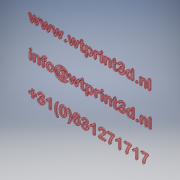
# Autodesk Inventor part: tekst
Saved by Autodesk Inventor 2019.4 (Build 234330000, 330)
## iProperties
Created: 2020-06-08
Part Number: tekst
Material: Generic
Document SubType Name: Modeling
Designer: Jaap Kort
Density: 1 g/cm^3
Appearance: Dark Red
Author: Jaap Kort
Autodesk Inventor part; units mm, degrees
(part 1 of 2)
ref_plane "YZ Plane" through (0, 0, 0) normal (1, 0, 0) x (0, 1, 0)
ref_plane "XZ Plane" through (0, 0, 0) normal (0, 1, 0) x (-1, 0, 0)
ref_plane "XY Plane" through (0, 0, 0) normal (0, 0, 1) x (1, 0, 0)
sketch "Sketch1" plane through (0, 0, 0) normal (0, 0, 1) x (1, 0, 0)
  line L0 (0, 0) -> (85, 0) construction
  line L1 (85, 0) -> (85, 50) construction
  line L2 (85, 50) -> (0, 50) construction
  line L3 (0, 50) -> (0, 0) construction
  line L4 (5.8901, 47.723) -> (80.1344, 47.723) construction
  line L5 (80.1344, 47.723) -> (80.1344, 6.1788) construction
  line L6 (80.1344, 6.1788) -> (5.8901, 6.1788) construction
  line L7 (5.8901, 6.1788) -> (5.8901, 47.723) construction
  line L8 (7.2722, 45.4071) -> (7.887, 43.082)
  line L9 (7.887, 43.082) -> (8.4417, 45.2407)
  spline S0 degree 2 poles (8.4417, 45.2407) (8.5434, 45.5874) (8.6543, 45.8694) (8.964, 46.1329) (9.2275, 46.1329) knots 0 0 0 1 2 3 3 3
  spline S1 degree 2 poles (9.2275, 46.1329) (9.4956, 46.1329) (9.8099, 45.8694) (9.9255, 45.5782) (10.0133, 45.2823) knots 0 0 0 1 2 3 3 3
  line L10 (10.0133, 45.2823) -> (10.5819, 43.082)
  line L11 (10.5819, 43.082) -> (11.2152, 45.4395)
  spline S2 degree 2 poles (11.2152, 45.4395) (11.2753, 45.666) (11.3677, 45.9202) (11.6127, 46.1329) (11.8346, 46.1329) knots 0 0 0 1 2 3 3 3
  spline S3 degree 2 poles (11.8346, 46.1329) (12.0611, 46.1329) (12.3939, 45.8185) (12.3939, 45.6059) knots 0 0 0 1 2 2 2
  spline S4 degree 2 poles (12.3939, 45.6059) (12.3939, 45.4303) (12.2599, 45.0605) knots 0 0 0 1 1 1
  line L12 (12.2599, 45.0605) -> (11.377, 42.4672)
  spline S5 degree 2 poles (11.377, 42.4672) (11.2799, 42.2038) (11.1458, 41.8848) (10.8408, 41.6259) (10.5727, 41.6259) knots 0 0 0 1 2 3 3 3
  spline S6 degree 2 poles (10.5727, 41.6259) (10.2953, 41.6259) (9.981, 41.8987) (9.8377, 42.2823) (9.7637, 42.5366) knots 0 0 0 1 2 3 3 3
  line L13 (9.7637, 42.5366) -> (9.2275, 44.5843)
  line L14 (9.2275, 44.5843) -> (8.7098, 42.5366)
  spline S7 degree 2 poles (8.7098, 42.5366) (8.5942, 42.1159) (8.2938, 41.6259) (7.9009, 41.6259) knots 0 0 0 1 2 2 2
  spline S8 degree 2 poles (7.9009, 41.6259) (7.7021, 41.6259) (7.4201, 41.7831) (7.2352, 42.0651) (7.1197, 42.3887) (7.0734, 42.5227) knots 0 0 0 1 2 3 4 4 4
  line L15 (7.0734, 42.5227) -> (6.2136, 45.0605)
  spline S9 degree 2 poles (6.2136, 45.0605) (6.075, 45.4534) (6.075, 45.6059) knots 0 0 0 1 1 1
  spline S10 degree 2 poles (6.075, 45.6059) (6.075, 45.8139) (6.3939, 46.1329) (6.6343, 46.1329) knots 0 0 0 1 2 2 2
  spline S11 degree 2 poles (6.6343, 46.1329) (6.944, 46.1329) (7.1613, 45.7816) (7.2722, 45.4071) knots 0 0 0 1 2 2 2
  line L16 (13.9286, 45.4071) -> (14.5434, 43.082)
  line L17 (14.5434, 43.082) -> (15.0981, 45.2407)
  spline S12 degree 2 poles (15.0981, 45.2407) (15.1998, 45.5874) (15.3107, 45.8694) (15.6204, 46.1329) (15.8839, 46.1329) knots 0 0 0 1 2 3 3 3
  spline S13 degree 2 poles (15.8839, 46.1329) (16.152, 46.1329) (16.4663, 45.8694) (16.5819, 45.5782) (16.6697, 45.2823) knots 0 0 0 1 2 3 3 3
  line L18 (16.6697, 45.2823) -> (17.2383, 43.082)
  line L19 (17.2383, 43.082) -> (17.8716, 45.4395)
  spline S14 degree 2 poles (17.8716, 45.4395) (17.9317, 45.666) (18.0241, 45.9202) (18.2691, 46.1329) (18.491, 46.1329) knots 0 0 0 1 2 3 3 3
  spline S15 degree 2 poles (18.491, 46.1329) (18.7175, 46.1329) (19.0503, 45.8185) (19.0503, 45.6059) knots 0 0 0 1 2 2 2
  spline S16 degree 2 poles (19.0503, 45.6059) (19.0503, 45.4303) (18.9163, 45.0605) knots 0 0 0 1 1 1
  line L20 (18.9163, 45.0605) -> (18.0334, 42.4672)
  spline S17 degree 2 poles (18.0334, 42.4672) (17.9363, 42.2038) (17.8022, 41.8848) (17.4972, 41.6259) (17.2291, 41.6259) knots 0 0 0 1 2 3 3 3
  spline S18 degree 2 poles (17.2291, 41.6259) (16.9517, 41.6259) (16.6374, 41.8987) (16.4941, 42.2823) (16.4201, 42.5366) knots 0 0 0 1 2 3 3 3
  line L21 (16.4201, 42.5366) -> (15.8839, 44.5843)
  line L22 (15.8839, 44.5843) -> (15.3662, 42.5366)
  spline S19 degree 2 poles (15.3662, 42.5366) (15.2506, 42.1159) (14.9502, 41.6259) (14.5572, 41.6259) knots 0 0 0 1 2 2 2
  spline S20 degree 2 poles (14.5572, 41.6259) (14.3585, 41.6259) (14.0765, 41.7831) (13.8916, 42.0651) (13.776, 42.3887) (13.7298, 42.5227) knots 0 0 0 1 2 3 4 4 4
  line L23 (13.7298, 42.5227) -> (12.87, 45.0605)
  spline S21 degree 2 poles (12.87, 45.0605) (12.7314, 45.4534) (12.7314, 45.6059) knots 0 0 0 1 1 1
  spline S22 degree 2 poles (12.7314, 45.6059) (12.7314, 45.8139) (13.0503, 46.1329) (13.2907, 46.1329) knots 0 0 0 1 2 2 2
  spline S23 degree 2 poles (13.2907, 46.1329) (13.6004, 46.1329) (13.8176, 45.7816) (13.9286, 45.4071) knots 0 0 0 1 2 2 2
  line L24 (20.585, 45.4071) -> (21.1998, 43.082)
  line L25 (21.1998, 43.082) -> (21.7545, 45.2407)
  spline S24 degree 2 poles (21.7545, 45.2407) (21.8562, 45.5874) (21.9671, 45.8694) (22.2768, 46.1329) (22.5403, 46.1329) knots 0 0 0 1 2 3 3 3
  spline S25 degree 2 poles (22.5403, 46.1329) (22.8084, 46.1329) (23.1227, 45.8694) (23.2383, 45.5782) (23.3261, 45.2823) knots 0 0 0 1 2 3 3 3
  line L26 (23.3261, 45.2823) -> (23.8947, 43.082)
  line L27 (23.8947, 43.082) -> (24.528, 45.4395)
  spline S26 degree 2 poles (24.528, 45.4395) (24.5881, 45.666) (24.6805, 45.9202) (24.9255, 46.1329) (25.1474, 46.1329) knots 0 0 0 1 2 3 3 3
  spline S27 degree 2 poles (25.1474, 46.1329) (25.3739, 46.1329) (25.7067, 45.8185) (25.7067, 45.6059) knots 0 0 0 1 2 2 2
  spline S28 degree 2 poles (25.7067, 45.6059) (25.7067, 45.4303) (25.5727, 45.0605) knots 0 0 0 1 1 1
  line L28 (25.5727, 45.0605) -> (24.6898, 42.4672)
  spline S29 degree 2 poles (24.6898, 42.4672) (24.5927, 42.2038) (24.4586, 41.8848) (24.1536, 41.6259) (23.8854, 41.6259) knots 0 0 0 1 2 3 3 3
  spline S30 degree 2 poles (23.8854, 41.6259) (23.6081, 41.6259) (23.2938, 41.8987) (23.1505, 42.2823) (23.0765, 42.5366) knots 0 0 0 1 2 3 3 3
  line L29 (23.0765, 42.5366) -> (22.5403, 44.5843)
  line L30 (22.5403, 44.5843) -> (22.0226, 42.5366)
  spline S31 degree 2 poles (22.0226, 42.5366) (21.907, 42.1159) (21.6066, 41.6259) (21.2136, 41.6259) knots 0 0 0 1 2 2 2
  spline S32 degree 2 poles (21.2136, 41.6259) (21.0149, 41.6259) (20.7329, 41.7831) (20.548, 42.0651) (20.4324, 42.3887) (20.3862, 42.5227) knots 0 0 0 1 2 3 4 4 4
  line L31 (20.3862, 42.5227) -> (19.5264, 45.0605)
  spline S33 degree 2 poles (19.5264, 45.0605) (19.3878, 45.4534) (19.3878, 45.6059) knots 0 0 0 1 1 1
  spline S34 degree 2 poles (19.3878, 45.6059) (19.3878, 45.8139) (19.7067, 46.1329) (19.9471, 46.1329) knots 0 0 0 1 2 2 2
  spline S35 degree 2 poles (19.9471, 46.1329) (20.2568, 46.1329) (20.474, 45.7816) (20.585, 45.4071) knots 0 0 0 1 2 2 2
  spline S36 degree 2 poles (27.2044, 41.6259) (26.927, 41.6259) (26.5249, 41.9865) (26.5249, 42.3054) knots 0 0 0 1 2 2 2
  spline S37 degree 2 poles (26.5249, 42.3054) (26.5249, 42.5736) (26.9086, 42.9665) (27.1905, 42.9665) knots 0 0 0 1 2 2 2
  spline S38 degree 2 poles (27.1905, 42.9665) (27.4725, 42.9665) (27.87, 42.5782) (27.87, 42.3054) knots 0 0 0 1 2 2 2
  spline S39 degree 2 poles (27.87, 42.3054) (27.87, 41.9911) (27.4725, 41.6259) (27.2044, 41.6259) knots 0 0 0 1 2 2 2
  line L32 (29.8069, 45.4071) -> (30.4217, 43.082)
  line L33 (30.4217, 43.082) -> (30.9764, 45.2407)
  spline S40 degree 2 poles (30.9764, 45.2407) (31.078, 45.5874) (31.189, 45.8694) (31.4987, 46.1329) (31.7622, 46.1329) knots 0 0 0 1 2 3 3 3
  spline S41 degree 2 poles (31.7622, 46.1329) (32.0303, 46.1329) (32.3446, 45.8694) (32.4602, 45.5782) (32.548, 45.2823) knots 0 0 0 1 2 3 3 3
  line L34 (32.548, 45.2823) -> (33.1166, 43.082)
  line L35 (33.1166, 43.082) -> (33.7499, 45.4395)
  spline S42 degree 2 poles (33.7499, 45.4395) (33.8099, 45.666) (33.9024, 45.9202) (34.1474, 46.1329) (34.3693, 46.1329) knots 0 0 0 1 2 3 3 3
  spline S43 degree 2 poles (34.3693, 46.1329) (34.5958, 46.1329) (34.9286, 45.8185) (34.9286, 45.6059) knots 0 0 0 1 2 2 2
  spline S44 degree 2 poles (34.9286, 45.6059) (34.9286, 45.4303) (34.7945, 45.0605) knots 0 0 0 1 1 1
  line L36 (34.7945, 45.0605) -> (33.9116, 42.4672)
  spline S45 degree 2 poles (33.9116, 42.4672) (33.8146, 42.2038) (33.6805, 41.8848) (33.3754, 41.6259) (33.1073, 41.6259) knots 0 0 0 1 2 3 3 3
  spline S46 degree 2 poles (33.1073, 41.6259) (32.83, 41.6259) (32.5156, 41.8987) (32.3723, 42.2823) (32.2984, 42.5366) knots 0 0 0 1 2 3 3 3
  line L37 (32.2984, 42.5366) -> (31.7622, 44.5843)
  line L38 (31.7622, 44.5843) -> (31.2445, 42.5366)
  spline S47 degree 2 poles (31.2445, 42.5366) (31.1289, 42.1159) (30.8284, 41.6259) (30.4355, 41.6259) knots 0 0 0 1 2 2 2
  spline S48 degree 2 poles (30.4355, 41.6259) (30.2368, 41.6259) (29.9548, 41.7831) (29.7699, 42.0651) (29.6543, 42.3887) (29.6081, 42.5227) knots 0 0 0 1 2 3 4 4 4
  line L39 (29.6081, 42.5227) -> (28.7483, 45.0605)
  spline S49 degree 2 poles (28.7483, 45.0605) (28.6096, 45.4534) (28.6096, 45.6059) knots 0 0 0 1 1 1
  spline S50 degree 2 poles (28.6096, 45.6059) (28.6096, 45.8139) (28.9286, 46.1329) (29.169, 46.1329) knots 0 0 0 1 2 2 2
  spline S51 degree 2 poles (29.169, 46.1329) (29.4787, 46.1329) (29.6959, 45.7816) (29.8069, 45.4071) knots 0 0 0 1 2 2 2
  line L40 (35.7791, 46.0404) -> (35.8115, 46.0404)
  line L41 (35.8115, 46.0404) -> (35.8115, 46.6044)
  spline S52 degree 2 poles (35.8115, 46.6044) (35.8115, 46.8679) (35.8392, 47.1776) (35.9317, 47.3301) knots 0 0 0 1 2 2 2
  spline S53 degree 2 poles (35.9317, 47.3301) (35.9825, 47.4272) (36.2599, 47.5843) (36.4263, 47.5843) knots 0 0 0 1 2 2 2
  spline S54 degree 2 poles (36.4263, 47.5843) (36.662, 47.5843) (36.8515, 47.4087) knots 0 0 0 1 1 1
  spline S55 degree 2 poles (36.8515, 47.4087) (36.981, 47.2885) (37.0457, 46.9603) (37.0457, 46.6876) knots 0 0 0 1 2 2 2
  line L42 (37.0457, 46.6876) -> (37.0457, 46.0404)
  line L43 (37.0457, 46.0404) -> (37.3554, 46.0404)
  spline S56 degree 2 poles (37.3554, 46.0404) (37.6143, 46.0404) (37.9055, 45.7769) (37.9055, 45.5782) knots 0 0 0 1 2 2 2
  spline S57 degree 2 poles (37.9055, 45.5782) (37.9055, 45.3101) (37.4987, 45.1067) (37.1613, 45.1067) knots 0 0 0 1 2 2 2
  line L44 (37.1613, 45.1067) -> (37.0457, 45.1067)
  line L45 (37.0457, 45.1067) -> (37.0457, 43.2207)
  spline S58 degree 2 poles (37.0457, 43.2207) (37.0457, 42.9711) (37.078, 42.7307) (37.189, 42.6105) (37.323, 42.6105) knots 0 0 0 1 2 3 3 3
  spline S59 degree 2 poles (37.323, 42.6105) (37.4109, 42.6105) (37.7344, 42.6752) (37.8269, 42.6752) knots 0 0 0 1 2 2 2
  spline S60 degree 2 poles (37.8269, 42.6752) (37.9933, 42.6752) (38.2475, 42.421) (38.2475, 42.2407) knots 0 0 0 1 2 2 2
  spline S61 degree 2 poles (38.2475, 42.2407) (38.2475, 41.931) (37.6189, 41.6259) (37.0734, 41.6259) knots 0 0 0 1 2 2 2
  spline S62 degree 2 poles (37.0734, 41.6259) (36.5465, 41.6259) (35.9825, 41.9911) (35.8115, 42.629) (35.8115, 43.1375) knots 0 0 0 1 2 3 3 3
  line L46 (35.8115, 43.1375) -> (35.8115, 45.1067)
  line L47 (35.8115, 45.1067) -> (35.756, 45.1067)
  spline S63 degree 2 poles (35.756, 45.1067) (35.4879, 45.1067) (35.1967, 45.3702) (35.1967, 45.5782) knots 0 0 0 1 2 2 2
  spline S64 degree 2 poles (35.1967, 45.5782) (35.1967, 45.7816) (35.5018, 46.0404) (35.7791, 46.0404) knots 0 0 0 1 2 2 2
  line L48 (39.6851, 45.4534) -> (39.6851, 45.4071)
  spline S65 degree 2 poles (39.6851, 45.4071) (39.8469, 45.7585) (40.5311, 46.1236) (40.9656, 46.1236) knots 0 0 0 1 2 2 2
  spline S66 degree 2 poles (40.9656, 46.1236) (41.4787, 46.1236) (42.3523, 45.5874) (42.8515, 44.5751) (42.8515, 43.891) knots 0 0 0 1 2 3 3 3
  spline S67 degree 2 poles (42.8515, 43.891) (42.8515, 43.3825) (42.565, 42.5273) (42.0565, 41.9403) (41.3631, 41.6259) (40.9656, 41.6259) knots 0 0 0 1 2 3 4 4 4
  spline S68 degree 2 poles (40.9656, 41.6259) (40.4802, 41.6259) (39.8284, 42.0096) (39.6851, 42.3471) knots 0 0 0 1 2 2 2
  line L49 (39.6851, 42.3471) -> (39.6851, 40.8263)
  spline S69 degree 2 poles (39.6851, 40.8263) (39.6851, 40.0404) (39.0888, 40.0404) knots 0 0 0 1 1 1
  spline S70 degree 2 poles (39.0888, 40.0404) (38.7329, 40.0404) (38.5064, 40.4657) (38.5064, 40.8355) knots 0 0 0 1 2 2 2
  line L50 (38.5064, 40.8355) -> (38.5064, 45.4441)
  spline S71 degree 2 poles (38.5064, 45.4441) (38.5064, 45.7816) (38.8161, 46.1329) (39.0888, 46.1329) knots 0 0 0 1 2 2 2
  spline S72 degree 2 poles (39.0888, 46.1329) (39.3523, 46.1329) (39.6851, 45.7723) (39.6851, 45.4534) knots 0 0 0 1 2 2 2
  spline S73 degree 2 poles (41.6127, 43.9002) (41.6127, 44.3024) (41.3723, 44.8709) (40.9517, 45.1714) (40.7021, 45.1714) knots 0 0 0 1 2 3 3 3
  spline S74 degree 2 poles (40.7021, 45.1714) (40.2999, 45.1714) (39.736, 44.5242) (39.736, 43.8817) knots 0 0 0 1 2 2 2
  spline S75 degree 2 poles (39.736, 43.8817) (39.736, 43.2669) (40.2953, 42.6105) (40.7021, 42.6105) knots 0 0 0 1 2 2 2
  spline S76 degree 2 poles (40.7021, 42.6105) (40.9425, 42.6105) (41.3539, 42.8925) (41.6127, 43.4749) (41.6127, 43.9002) knots 0 0 0 1 2 3 3 3
  line L51 (44.8762, 43.2531) -> (44.8762, 42.3609)
  spline S77 degree 2 poles (44.8762, 42.3609) (44.8762, 42.0004) (44.5249, 41.6259) (44.2522, 41.6259) knots 0 0 0 1 2 2 2
  spline S78 degree 2 poles (44.2522, 41.6259) (43.9841, 41.6259) (43.642, 42.005) (43.642, 42.3609) knots 0 0 0 1 2 2 2
  line L52 (43.642, 42.3609) -> (43.642, 45.3332)
  spline S79 degree 2 poles (43.642, 45.3332) (43.642, 46.1329) (44.2475, 46.1329) knots 0 0 0 1 1 1
  spline S80 degree 2 poles (44.2475, 46.1329) (44.5572, 46.1329) (44.8254, 45.7446) (44.83, 45.4719) knots 0 0 0 1 2 2 2
  spline S81 degree 2 poles (44.83, 45.4719) (44.8854, 45.7677) (45.32, 46.1329) (45.6898, 46.1329) knots 0 0 0 1 2 2 2
  spline S82 degree 2 poles (45.6898, 46.1329) (46.0457, 46.1329) (46.7437, 45.7631) (46.7437, 45.4395) knots 0 0 0 1 2 2 2
  spline S83 degree 2 poles (46.7437, 45.4395) (46.7437, 45.2084) (46.4247, 44.9079) (46.2352, 44.9079) knots 0 0 0 1 2 2 2
  spline S84 degree 2 poles (46.2352, 44.9079) (46.1613, 44.9079) (45.7129, 45.0512) (45.5511, 45.0512) knots 0 0 0 1 2 2 2
  spline S85 degree 2 poles (45.5511, 45.0512) (45.3477, 45.0512) (45.0888, 44.8386) (44.9363, 44.3856) (44.8762, 43.7384) (44.8762, 43.2531) knots 0 0 0 1 2 3 4 4 4
  line L53 (48.4725, 45.4487) -> (48.4725, 42.3609)
  spline S86 degree 2 poles (48.4725, 42.3609) (48.4725, 42.005) (48.1212, 41.6259) (47.8485, 41.6259) knots 0 0 0 1 2 2 2
  spline S87 degree 2 poles (47.8485, 41.6259) (47.5757, 41.6259) (47.2383, 42.0142) (47.2383, 42.3609) knots 0 0 0 1 2 2 2
  line L54 (47.2383, 42.3609) -> (47.2383, 45.4164)
  spline S88 degree 2 poles (47.2383, 45.4164) (47.2383, 45.7631) (47.5757, 46.1329) (47.8485, 46.1329) knots 0 0 0 1 2 2 2
  spline S89 degree 2 poles (47.8485, 46.1329) (48.1212, 46.1329) (48.4725, 45.7631) (48.4725, 45.4487) knots 0 0 0 1 2 2 2
  spline S90 degree 2 poles (47.8623, 46.4703) (47.6081, 46.4703) (47.2383, 46.7893) (47.2383, 47.0759) knots 0 0 0 1 2 2 2
  spline S91 degree 2 poles (47.2383, 47.0759) (47.2383, 47.3393) (47.6127, 47.6768) (47.8623, 47.6768) knots 0 0 0 1 2 2 2
  spline S92 degree 2 poles (47.8623, 47.6768) (48.0981, 47.6768) (48.4725, 47.3671) (48.4725, 47.0759) knots 0 0 0 1 2 2 2
  spline S93 degree 2 poles (48.4725, 47.0759) (48.4725, 46.7939) (48.1073, 46.4703) (47.8623, 46.4703) knots 0 0 0 1 2 2 2
  line L55 (50.5989, 45.4672) -> (50.5989, 45.421)
  spline S94 degree 2 poles (50.5989, 45.421) (50.7375, 45.7677) (51.4448, 46.1329) (51.9024, 46.1329) knots 0 0 0 1 2 2 2
  spline S95 degree 2 poles (51.9024, 46.1329) (52.3462, 46.1329) (53.0534, 45.7446) (53.2291, 45.3887) knots 0 0 0 1 2 2 2
  spline S96 degree 2 poles (53.2291, 45.3887) (53.34, 45.1806) (53.4047, 44.7045) (53.4047, 44.3486) knots 0 0 0 1 2 2 2
  line L56 (53.4047, 44.3486) -> (53.4047, 42.3609)
  spline S97 degree 2 poles (53.4047, 42.3609) (53.4047, 42.005) (53.0673, 41.6259) (52.7945, 41.6259) knots 0 0 0 1 2 2 2
  spline S98 degree 2 poles (52.7945, 41.6259) (52.5172, 41.6259) (52.1751, 42.0142) (52.1751, 42.3609) knots 0 0 0 1 2 2 2
  line L57 (52.1751, 42.3609) -> (52.1751, 44.1406)
  spline S99 degree 2 poles (52.1751, 44.1406) (52.1751, 44.6491) (51.9116, 45.1483) (51.5234, 45.1483) knots 0 0 0 1 2 2 2
  spline S100 degree 2 poles (51.5234, 45.1483) (51.2645, 45.1483) (50.8392, 44.8386) (50.7237, 44.5289) knots 0 0 0 1 2 2 2
  spline S101 degree 2 poles (50.7237, 44.5289) (50.6636, 44.344) (50.6636, 43.7014) knots 0 0 0 1 1 1
  line L58 (50.6636, 43.7014) -> (50.6636, 42.3609)
  spline S102 degree 2 poles (50.6636, 42.3609) (50.6636, 42.0004) (50.3169, 41.6259) (50.0395, 41.6259) knots 0 0 0 1 2 2 2
  spline S103 degree 2 poles (50.0395, 41.6259) (49.7714, 41.6259) (49.4294, 42.0142) (49.4294, 42.3609) knots 0 0 0 1 2 2 2
  line L59 (49.4294, 42.3609) -> (49.4294, 45.4487)
  spline S104 degree 2 poles (49.4294, 45.4487) (49.4294, 45.7816) (49.7391, 46.1329) (50.0072, 46.1329) knots 0 0 0 1 2 2 2
  spline S105 degree 2 poles (50.0072, 46.1329) (50.1736, 46.1329) (50.4417, 45.9757) (50.5989, 45.6706) (50.5989, 45.4672) knots 0 0 0 1 2 3 3 3
  line L60 (54.5511, 46.0404) -> (54.5834, 46.0404)
  line L61 (54.5834, 46.0404) -> (54.5834, 46.6044)
  spline S106 degree 2 poles (54.5834, 46.6044) (54.5834, 46.8679) (54.6112, 47.1776) (54.7036, 47.3301) knots 0 0 0 1 2 2 2
  spline S107 degree 2 poles (54.7036, 47.3301) (54.7545, 47.4272) (55.0318, 47.5843) (55.1982, 47.5843) knots 0 0 0 1 2 2 2
  spline S108 degree 2 poles (55.1982, 47.5843) (55.434, 47.5843) (55.6235, 47.4087) knots 0 0 0 1 1 1
  spline S109 degree 2 poles (55.6235, 47.4087) (55.7529, 47.2885) (55.8176, 46.9603) (55.8176, 46.6876) knots 0 0 0 1 2 2 2
  line L62 (55.8176, 46.6876) -> (55.8176, 46.0404)
  line L63 (55.8176, 46.0404) -> (56.1274, 46.0404)
  spline S110 degree 2 poles (56.1274, 46.0404) (56.3862, 46.0404) (56.6774, 45.7769) (56.6774, 45.5782) knots 0 0 0 1 2 2 2
  spline S111 degree 2 poles (56.6774, 45.5782) (56.6774, 45.3101) (56.2707, 45.1067) (55.9332, 45.1067) knots 0 0 0 1 2 2 2
  line L64 (55.9332, 45.1067) -> (55.8176, 45.1067)
  line L65 (55.8176, 45.1067) -> (55.8176, 43.2207)
  spline S112 degree 2 poles (55.8176, 43.2207) (55.8176, 42.9711) (55.85, 42.7307) (55.9609, 42.6105) (56.095, 42.6105) knots 0 0 0 1 2 3 3 3
  spline S113 degree 2 poles (56.095, 42.6105) (56.1828, 42.6105) (56.5064, 42.6752) (56.5989, 42.6752) knots 0 0 0 1 2 2 2
  spline S114 degree 2 poles (56.5989, 42.6752) (56.7653, 42.6752) (57.0195, 42.421) (57.0195, 42.2407) knots 0 0 0 1 2 2 2
  spline S115 degree 2 poles (57.0195, 42.2407) (57.0195, 41.931) (56.3908, 41.6259) (55.8454, 41.6259) knots 0 0 0 1 2 2 2
  spline S116 degree 2 poles (55.8454, 41.6259) (55.3184, 41.6259) (54.7545, 41.9911) (54.5834, 42.629) (54.5834, 43.1375) knots 0 0 0 1 2 3 3 3
  line L66 (54.5834, 43.1375) -> (54.5834, 45.1067)
  line L67 (54.5834, 45.1067) -> (54.528, 45.1067)
  spline S117 degree 2 poles (54.528, 45.1067) (54.2599, 45.1067) (53.9687, 45.3702) (53.9687, 45.5782) knots 0 0 0 1 2 2 2
  spline S118 degree 2 poles (53.9687, 45.5782) (53.9687, 45.7816) (54.2737, 46.0404) (54.5511, 46.0404) knots 0 0 0 1 2 2 2
  spline S119 degree 2 poles (59.0303, 45.3517) (59.3585, 45.3517) (59.83, 45.7307) (59.83, 46.0913) knots 0 0 0 1 2 2 2
  spline S120 degree 2 poles (59.83, 46.0913) (59.83, 46.3548) (59.4602, 46.743) (59.1458, 46.743) knots 0 0 0 1 2 2 2
  spline S121 degree 2 poles (59.1458, 46.743) (58.924, 46.743) (58.6466, 46.6229) (58.4895, 46.4333) (58.3138, 46.0543) (58.263, 45.9434) knots 0 0 0 1 2 3 4 4 4
  spline S122 degree 2 poles (58.263, 45.9434) (58.2121, 45.8278) (57.9671, 45.7169) (57.8146, 45.7169) knots 0 0 0 1 2 2 2
  spline S123 degree 2 poles (57.8146, 45.7169) (57.6204, 45.7169) (57.3107, 46.0219) (57.3107, 46.2669) knots 0 0 0 1 2 2 2
  spline S124 degree 2 poles (57.3107, 46.2669) (57.3107, 46.4934) (57.5742, 46.9695) (58.0734, 47.3948) (58.8038, 47.6537) (59.2522, 47.6537) knots 0 0 0 1 2 3 4 4 4
  spline S125 degree 2 poles (59.2522, 47.6537) (59.6451, 47.6537) (60.3015, 47.4364) (60.7915, 47.0204) (61.0411, 46.4749) (61.0411, 46.1606) knots 0 0 0 1 2 3 4 4 4
  spline S126 degree 2 poles (61.0411, 46.1606) (61.0411, 45.7492) (60.6805, 45.1529) (60.3847, 44.9541) knots 0 0 0 1 2 2 2
  spline S127 degree 2 poles (60.3847, 44.9541) (60.6574, 44.8432) (61.0965, 44.3994) (61.3184, 43.8586) (61.3184, 43.5443) knots 0 0 0 1 2 3 3 3
  spline S128 degree 2 poles (61.3184, 43.5443) (61.3184, 43.1745) (61.018, 42.4765) (60.4401, 41.931) (59.6451, 41.6259) (59.169, 41.6259) knots 0 0 0 1 2 3 4 4 4
  spline S129 degree 2 poles (59.169, 41.6259) (58.679, 41.6259) (57.9024, 41.9773) (57.4032, 42.5042) (57.1443, 43.0728) (57.1443, 43.2669) knots 0 0 0 1 2 3 4 4 4
  spline S130 degree 2 poles (57.1443, 43.2669) (57.1443, 43.5304) (57.4864, 43.854) (57.7406, 43.854) knots 0 0 0 1 2 2 2
  spline S131 degree 2 poles (57.7406, 43.854) (57.8747, 43.854) (58.1197, 43.6922) (58.1659, 43.5489) knots 0 0 0 1 2 2 2
  spline S132 degree 2 poles (58.1659, 43.5489) (58.36, 43.0497) (58.7899, 42.5597) (59.1782, 42.5597) knots 0 0 0 1 2 2 2
  spline S133 degree 2 poles (59.1782, 42.5597) (59.4001, 42.5597) (59.8069, 42.7769) (60.0796, 43.2115) (60.0796, 43.4981) knots 0 0 0 1 2 3 3 3
  spline S134 degree 2 poles (60.0796, 43.4981) (60.0796, 43.9233) (59.622, 44.3948) (59.2152, 44.3948) knots 0 0 0 1 2 2 2
  spline S135 degree 2 poles (59.2152, 44.3948) (59.1458, 44.3948) (58.8177, 44.3625) (58.7622, 44.3625) knots 0 0 0 1 2 2 2
  spline S136 degree 2 poles (58.7622, 44.3625) (58.5126, 44.3625) (58.226, 44.6213) (58.226, 44.8524) knots 0 0 0 1 2 2 2
  spline S137 degree 2 poles (58.226, 44.8524) (58.226, 45.0789) (58.5634, 45.3517) (58.8685, 45.3517) knots 0 0 0 1 2 2 2
  line L68 (58.8685, 45.3517) -> (59.0303, 45.3517)
  line L69 (65.0996, 42.3193) -> (65.0996, 42.3378)
  spline S138 degree 2 poles (65.0996, 42.3378) (65.0257, 42.1159) (64.5865, 41.7924) (64.0734, 41.6259) (63.7683, 41.6259) knots 0 0 0 1 2 3 3 3
  spline S139 degree 2 poles (63.7683, 41.6259) (63.3616, 41.6259) (62.6774, 41.968) (62.1782, 42.5967) (61.924, 43.4333) (61.924, 43.9233) knots 0 0 0 1 2 3 4 4 4
  spline S140 degree 2 poles (61.924, 43.9233) (61.924, 44.9541) (62.9455, 46.1236) (63.7868, 46.1236) knots 0 0 0 1 2 2 2
  spline S141 degree 2 poles (63.7868, 46.1236) (64.2676, 46.1236) (64.9332, 45.7908) (65.0996, 45.4811) knots 0 0 0 1 2 2 2
  line L70 (65.0996, 45.4811) -> (65.0996, 46.9788)
  spline S142 degree 2 poles (65.0996, 46.9788) (65.0996, 47.3347) (65.4047, 47.723) (65.6913, 47.723) knots 0 0 0 1 2 2 2
  spline S143 degree 2 poles (65.6913, 47.723) (65.9687, 47.723) (66.2784, 47.3625) (66.2784, 47.0343) knots 0 0 0 1 2 2 2
  line L71 (66.2784, 47.0343) -> (66.2784, 42.3193)
  spline S144 degree 2 poles (66.2784, 42.3193) (66.2784, 41.9819) (65.9502, 41.6259) (65.6913, 41.6259) knots 0 0 0 1 2 2 2
  spline S145 degree 2 poles (65.6913, 41.6259) (65.4324, 41.6259) (65.0996, 41.9911) (65.0996, 42.3193) knots 0 0 0 1 2 2 2
  spline S146 degree 2 poles (63.1628, 43.8863) (63.1628, 43.4657) (63.417, 42.8925) (63.8469, 42.6105) (64.0965, 42.6105) knots 0 0 0 1 2 3 3 3
  spline S147 degree 2 poles (64.0965, 42.6105) (64.3554, 42.6105) (64.7807, 42.8786) (65.0395, 43.4518) (65.0395, 43.8863) knots 0 0 0 1 2 3 3 3
  spline S148 degree 2 poles (65.0395, 43.8863) (65.0395, 44.2931) (64.7807, 44.8756) (64.3462, 45.1714) (64.0919, 45.1714) knots 0 0 0 1 2 3 3 3
  spline S149 degree 2 poles (64.0919, 45.1714) (63.8238, 45.1714) (63.4032, 44.8663) (63.1628, 44.2839) (63.1628, 43.8863) knots 0 0 0 1 2 3 3 3
  spline S150 degree 2 poles (68.0811, 41.6259) (67.8038, 41.6259) (67.4016, 41.9865) (67.4016, 42.3054) knots 0 0 0 1 2 2 2
  spline S151 degree 2 poles (67.4016, 42.3054) (67.4016, 42.5736) (67.7853, 42.9665) (68.0673, 42.9665) knots 0 0 0 1 2 2 2
  spline S152 degree 2 poles (68.0673, 42.9665) (68.3492, 42.9665) (68.7468, 42.5782) (68.7468, 42.3054) knots 0 0 0 1 2 2 2
  spline S153 degree 2 poles (68.7468, 42.3054) (68.7468, 41.9911) (68.3492, 41.6259) (68.0811, 41.6259) knots 0 0 0 1 2 2 2
  line L72 (70.9933, 45.4672) -> (70.9933, 45.421)
  spline S154 degree 2 poles (70.9933, 45.421) (71.132, 45.7677) (71.8392, 46.1329) (72.2968, 46.1329) knots 0 0 0 1 2 2 2
  spline S155 degree 2 poles (72.2968, 46.1329) (72.7406, 46.1329) (73.4479, 45.7446) (73.6235, 45.3887) knots 0 0 0 1 2 2 2
  spline S156 degree 2 poles (73.6235, 45.3887) (73.7344, 45.1806) (73.7992, 44.7045) (73.7992, 44.3486) knots 0 0 0 1 2 2 2
  line L73 (73.7992, 44.3486) -> (73.7992, 42.3609)
  spline S157 degree 2 poles (73.7992, 42.3609) (73.7992, 42.005) (73.4617, 41.6259) (73.189, 41.6259) knots 0 0 0 1 2 2 2
  spline S158 degree 2 poles (73.189, 41.6259) (72.9116, 41.6259) (72.5696, 42.0142) (72.5696, 42.3609) knots 0 0 0 1 2 2 2
  line L74 (72.5696, 42.3609) -> (72.5696, 44.1406)
  spline S159 degree 2 poles (72.5696, 44.1406) (72.5696, 44.6491) (72.3061, 45.1483) (71.9178, 45.1483) knots 0 0 0 1 2 2 2
  spline S160 degree 2 poles (71.9178, 45.1483) (71.6589, 45.1483) (71.2337, 44.8386) (71.1181, 44.5289) knots 0 0 0 1 2 2 2
  spline S161 degree 2 poles (71.1181, 44.5289) (71.058, 44.344) (71.058, 43.7014) knots 0 0 0 1 1 1
  line L75 (71.058, 43.7014) -> (71.058, 42.3609)
  spline S162 degree 2 poles (71.058, 42.3609) (71.058, 42.0004) (70.7113, 41.6259) (70.434, 41.6259) knots 0 0 0 1 2 2 2
  spline S163 degree 2 poles (70.434, 41.6259) (70.1659, 41.6259) (69.8238, 42.0142) (69.8238, 42.3609) knots 0 0 0 1 2 2 2
  line L76 (69.8238, 42.3609) -> (69.8238, 45.4487)
  spline S164 degree 2 poles (69.8238, 45.4487) (69.8238, 45.7816) (70.1335, 46.1329) (70.4016, 46.1329) knots 0 0 0 1 2 2 2
  spline S165 degree 2 poles (70.4016, 46.1329) (70.568, 46.1329) (70.8361, 45.9757) (70.9933, 45.6706) (70.9933, 45.4672) knots 0 0 0 1 2 3 3 3
  line L77 (74.8022, 42.3609) -> (74.8022, 46.9927)
  spline S166 degree 2 poles (74.8022, 46.9927) (74.8022, 47.344) (75.1304, 47.723) (75.4124, 47.723) knots 0 0 0 1 2 2 2
  spline S167 degree 2 poles (75.4124, 47.723) (75.6944, 47.723) (76.0364, 47.3486) (76.0364, 46.9927) knots 0 0 0 1 2 2 2
  line L78 (76.0364, 46.9927) -> (76.0364, 42.3609)
  spline S168 degree 2 poles (76.0364, 42.3609) (76.0364, 42.0004) (75.6898, 41.6259) (75.4124, 41.6259) knots 0 0 0 1 2 2 2
  spline S169 degree 2 poles (75.4124, 41.6259) (75.1397, 41.6259) (74.8022, 42.0142) (74.8022, 42.3609) knots 0 0 0 1 2 2 2
  line L79 (7.679, 26.418) -> (7.679, 23.3301)
  spline S170 degree 2 poles (7.679, 23.3301) (7.679, 22.9742) (7.3277, 22.5952) (7.0549, 22.5952) knots 0 0 0 1 2 2 2
  spline S171 degree 2 poles (7.0549, 22.5952) (6.7822, 22.5952) (6.4448, 22.9835) (6.4448, 23.3301) knots 0 0 0 1 2 2 2
  line L80 (6.4448, 23.3301) -> (6.4448, 26.3856)
  spline S172 degree 2 poles (6.4448, 26.3856) (6.4448, 26.7323) (6.7822, 27.1021) (7.0549, 27.1021) knots 0 0 0 1 2 2 2
  spline S173 degree 2 poles (7.0549, 27.1021) (7.3277, 27.1021) (7.679, 26.7323) (7.679, 26.418) knots 0 0 0 1 2 2 2
  spline S174 degree 2 poles (7.0688, 27.4395) (6.8146, 27.4395) (6.4448, 27.7585) (6.4448, 28.0451) knots 0 0 0 1 2 2 2
  spline S175 degree 2 poles (6.4448, 28.0451) (6.4448, 28.3086) (6.8192, 28.646) (7.0688, 28.646) knots 0 0 0 1 2 2 2
  spline S176 degree 2 poles (7.0688, 28.646) (7.3046, 28.646) (7.679, 28.3363) (7.679, 28.0451) knots 0 0 0 1 2 2 2
  spline S177 degree 2 poles (7.679, 28.0451) (7.679, 27.7631) (7.3138, 27.4395) (7.0688, 27.4395) knots 0 0 0 1 2 2 2
  line L81 (9.8053, 26.4365) -> (9.8053, 26.3902)
  spline S178 degree 2 poles (9.8053, 26.3902) (9.944, 26.7369) (10.6512, 27.1021) (11.1089, 27.1021) knots 0 0 0 1 2 2 2
  spline S179 degree 2 poles (11.1089, 27.1021) (11.5526, 27.1021) (12.2599, 26.7138) (12.4355, 26.3579) knots 0 0 0 1 2 2 2
  spline S180 degree 2 poles (12.4355, 26.3579) (12.5465, 26.1499) (12.6112, 25.6737) (12.6112, 25.3178) knots 0 0 0 1 2 2 2
  line L82 (12.6112, 25.3178) -> (12.6112, 23.3301)
  spline S181 degree 2 poles (12.6112, 23.3301) (12.6112, 22.9742) (12.2737, 22.5952) (12.001, 22.5952) knots 0 0 0 1 2 2 2
  spline S182 degree 2 poles (12.001, 22.5952) (11.7237, 22.5952) (11.3816, 22.9835) (11.3816, 23.3301) knots 0 0 0 1 2 2 2
  line L83 (11.3816, 23.3301) -> (11.3816, 25.1098)
  spline S183 degree 2 poles (11.3816, 25.1098) (11.3816, 25.6183) (11.1181, 26.1175) (10.7298, 26.1175) knots 0 0 0 1 2 2 2
  spline S184 degree 2 poles (10.7298, 26.1175) (10.471, 26.1175) (10.0457, 25.8078) (9.9301, 25.4981) knots 0 0 0 1 2 2 2
  spline S185 degree 2 poles (9.9301, 25.4981) (9.87, 25.3132) (9.87, 24.6707) knots 0 0 0 1 1 1
  line L84 (9.87, 24.6707) -> (9.87, 23.3301)
  spline S186 degree 2 poles (9.87, 23.3301) (9.87, 22.9696) (9.5233, 22.5952) (9.246, 22.5952) knots 0 0 0 1 2 2 2
  spline S187 degree 2 poles (9.246, 22.5952) (8.9779, 22.5952) (8.6358, 22.9835) (8.6358, 23.3301) knots 0 0 0 1 2 2 2
  line L85 (8.6358, 23.3301) -> (8.6358, 26.418)
  spline S188 degree 2 poles (8.6358, 26.418) (8.6358, 26.7508) (8.9455, 27.1021) (9.2136, 27.1021) knots 0 0 0 1 2 2 2
  spline S189 degree 2 poles (9.2136, 27.1021) (9.3801, 27.1021) (9.6482, 26.9449) (9.8053, 26.6398) (9.8053, 26.4365) knots 0 0 0 1 2 3 3 3
  line L86 (13.6096, 27.0096) -> (13.7807, 27.0096)
  line L87 (13.7807, 27.0096) -> (13.7807, 27.25)
  spline S190 degree 2 poles (13.7807, 27.25) (13.7807, 27.7677) (14.0534, 28.401) (14.7052, 28.6922) (15.2506, 28.6922) knots 0 0 0 1 2 3 3 3
  spline S191 degree 2 poles (15.2506, 28.6922) (16.2722, 28.6922) (16.2722, 28.156) knots 0 0 0 1 1 1
  spline S192 degree 2 poles (16.2722, 28.156) (16.2722, 27.9757) (16.0272, 27.7123) (15.8608, 27.7123) knots 0 0 0 1 2 2 2
  spline S193 degree 2 poles (15.8608, 27.7123) (15.7822, 27.7123) (15.4771, 27.7585) (15.3847, 27.7585) knots 0 0 0 1 2 2 2
  spline S194 degree 2 poles (15.3847, 27.7585) (15.1489, 27.7585) (15.0149, 27.4858) (15.0149, 27.1853) knots 0 0 0 1 2 2 2
  line L88 (15.0149, 27.1853) -> (15.0149, 27.0096)
  line L89 (15.0149, 27.0096) -> (15.1952, 27.0096)
  spline S195 degree 2 poles (15.1952, 27.0096) (15.8885, 27.0096) (15.8885, 26.5613) knots 0 0 0 1 1 1
  spline S196 degree 2 poles (15.8885, 26.5613) (15.8885, 26.2469) (15.4956, 26.0759) (15.1952, 26.0759) knots 0 0 0 1 2 2 2
  line L90 (15.1952, 26.0759) -> (15.0149, 26.0759)
  line L91 (15.0149, 26.0759) -> (15.0149, 23.3301)
  spline S197 degree 2 poles (15.0149, 23.3301) (15.0149, 22.9788) (14.6682, 22.5952) (14.3908, 22.5952) knots 0 0 0 1 2 2 2
  spline S198 degree 2 poles (14.3908, 22.5952) (14.1274, 22.5952) (13.7807, 22.9788) (13.7807, 23.3301) knots 0 0 0 1 2 2 2
  line L92 (13.7807, 23.3301) -> (13.7807, 26.0759)
  line L93 (13.7807, 26.0759) -> (13.568, 26.0759)
  spline S199 degree 2 poles (13.568, 26.0759) (13.2999, 26.0759) (12.9902, 26.3348) (12.9902, 26.5474) knots 0 0 0 1 2 2 2
  spline S200 degree 2 poles (12.9902, 26.5474) (12.9902, 27.0096) (13.6096, 27.0096) knots 0 0 0 1 1 1
  spline S201 degree 2 poles (20.5064, 24.8509) (20.5064, 24.3563) (20.1967, 23.5243) (19.605, 22.9141) (18.7961, 22.5952) (18.2876, 22.5952) knots 0 0 0 1 2 3 4 4 4
  spline S202 degree 2 poles (18.2876, 22.5952) (17.7838, 22.5952) (16.9794, 22.9187) (16.3878, 23.5289) (16.0827, 24.3517) (16.0827, 24.8509) knots 0 0 0 1 2 3 4 4 4
  spline S203 degree 2 poles (16.0827, 24.8509) (16.0827, 25.3548) (16.3878, 26.1822) (16.9702, 26.7785) (17.7976, 27.1021) (18.2876, 27.1021) knots 0 0 0 1 2 3 4 4 4
  spline S204 degree 2 poles (18.2876, 27.1021) (18.7868, 27.1021) (19.6143, 26.7739) (20.2013, 26.1684) (20.5064, 25.3455) (20.5064, 24.8509) knots 0 0 0 1 2 3 4 4 4
  spline S205 degree 2 poles (19.2676, 24.8509) (19.2676, 25.475) (18.7314, 26.1499) (18.2876, 26.1499) knots 0 0 0 1 2 2 2
  spline S206 degree 2 poles (18.2876, 26.1499) (18.001, 26.1499) (17.5665, 25.854) (17.3215, 25.2577) (17.3215, 24.8509) knots 0 0 0 1 2 3 3 3
  spline S207 degree 2 poles (17.3215, 24.8509) (17.3215, 24.4442) (17.5619, 23.8525) (17.9918, 23.552) (18.2876, 23.552) knots 0 0 0 1 2 3 3 3
  spline S208 degree 2 poles (18.2876, 23.552) (18.7314, 23.552) (19.2676, 24.2315) (19.2676, 24.8509) knots 0 0 0 1 2 2 2
  line L94 (25.6466, 26.5659) -> (25.7113, 27.0004)
  line L95 (25.7113, 27.0004) -> (26.8993, 27.0004)
  line L96 (26.8993, 27.0004) -> (26.2891, 24.0512)
  spline S209 degree 2 poles (26.2891, 24.0512) (26.2475, 23.8432) (26.2475, 23.7647) knots 0 0 0 1 1 1
  spline S210 degree 2 poles (26.2475, 23.7647) (26.2475, 23.6999) (26.2938, 23.6491) (26.3169, 23.6491) knots 0 0 0 1 2 2 2
  spline S211 degree 2 poles (26.3169, 23.6491) (26.4972, 23.6491) (27.1304, 24.1714) (27.6112, 25.0913) (27.6112, 25.6368) knots 0 0 0 1 2 3 3 3
  spline S212 degree 2 poles (27.6112, 25.6368) (27.6112, 26.0898) (27.2691, 26.8895) (26.622, 27.4719) (25.6559, 27.8093) (25.0457, 27.8093) knots 0 0 0 1 2 3 4 4 4
  spline S213 degree 2 poles (25.0457, 27.8093) (24.4263, 27.8093) (23.3816, 27.4811) (22.6004, 26.8802) (22.3508, 26.5474) knots 0 0 0 1 2 3 3 3
  spline S214 degree 2 poles (22.3508, 26.5474) (22.1058, 26.0435) (21.8608, 25.1006) (21.8608, 24.6013) knots 0 0 0 1 2 2 2
  spline S215 degree 2 poles (21.8608, 24.6013) (21.8608, 23.9449) (22.3785, 22.8633) (23.3723, 22.1329) (24.7915, 21.8278) (25.679, 21.9157) knots 0 0 0 1 2 3 4 4 4
  spline S216 degree 2 poles (25.679, 21.9157) (26.4001, 21.9989) (27.3708, 22.4704) (27.736, 22.9234) knots 0 0 0 1 2 2 2
  line L97 (27.736, 22.9234) -> (28.6975, 22.9234)
  spline S217 degree 2 poles (28.6975, 22.9234) (28.4756, 22.3733) (27.8053, 21.703) (26.9039, 21.2408) (25.7992, 21.0004) (25.1474, 21.0004) knots 0 0 0 1 2 3 4 4 4
  spline S218 degree 2 poles (25.1474, 21.0004) (24.172, 21.0004) (22.5958, 21.5135) (21.5141, 22.4935) (20.964, 23.8386) (20.964, 24.6568) knots 0 0 0 1 2 3 4 4 4
  spline S219 degree 2 poles (20.964, 24.6568) (20.964, 25.5073) (21.5326, 26.9819) (22.6004, 28.0774) (24.1397, 28.6922) (25.0642, 28.6922) knots 0 0 0 1 2 3 4 4 4
  spline S220 degree 2 poles (25.0642, 28.6922) (25.8223, 28.6922) (27.0981, 28.2485) (28.0041, 27.4072) (28.4848, 26.2608) (28.4848, 25.5767) knots 0 0 0 1 2 3 4 4 4
  spline S221 degree 2 poles (28.4848, 25.5767) (28.4848, 25.0358) (28.0965, 23.9958) (27.3754, 23.173) (26.3955, 22.6922) (25.8269, 22.6922) knots 0 0 0 1 2 3 4 4 4
  spline S222 degree 2 poles (25.8269, 22.6922) (25.4848, 22.6922) (25.0873, 22.9372) (25.0549, 23.1406) knots 0 0 0 1 2 2 2
  spline S223 degree 2 poles (25.0549, 23.1406) (24.8007, 22.8124) (23.8623, 22.6275) (22.9887, 22.9835) (22.4478, 23.834) (22.4478, 24.4488) knots 0 0 0 1 2 3 4 4 4
  spline S224 degree 2 poles (22.4478, 24.4488) (22.4478, 25.0821) (22.9887, 26.3024) (24.0056, 27.0929) (24.6482, 27.0929) knots 0 0 0 1 2 3 3 3
  spline S225 degree 2 poles (24.6482, 27.0929) (25.4016, 27.0929) (25.6466, 26.5659) knots 0 0 0 1 1 1
  spline S226 degree 2 poles (23.6266, 24.458) (23.6266, 24.0143) (23.9779, 23.5659) (24.2506, 23.5659) knots 0 0 0 1 2 2 2
  spline S227 degree 2 poles (24.2506, 23.5659) (24.5834, 23.5659) (25.1058, 24.116) (25.3831, 24.9804) (25.3831, 25.3871) knots 0 0 0 1 2 3 3 3
  spline S228 degree 2 poles (25.3831, 25.3871) (25.3831, 25.5813) (25.2953, 25.891) (25.1243, 26.1129) (24.8885, 26.2238) (24.736, 26.2238) knots 0 0 0 1 2 3 4 4 4
  spline S229 degree 2 poles (24.736, 26.2238) (24.4263, 26.2238) (23.9132, 25.7246) (23.6266, 24.9018) (23.6266, 24.458) knots 0 0 0 1 2 3 3 3
  line L98 (30.1304, 26.3764) -> (30.7452, 24.0512)
  line L99 (30.7452, 24.0512) -> (31.2999, 26.21)
  spline S230 degree 2 poles (31.2999, 26.21) (31.4016, 26.5566) (31.5126, 26.8386) (31.8223, 27.1021) (32.0858, 27.1021) knots 0 0 0 1 2 3 3 3
  spline S231 degree 2 poles (32.0858, 27.1021) (32.3539, 27.1021) (32.6682, 26.8386) (32.7838, 26.5474) (32.8716, 26.2516) knots 0 0 0 1 2 3 3 3
  line L100 (32.8716, 26.2516) -> (33.4401, 24.0512)
  line L101 (33.4401, 24.0512) -> (34.0734, 26.4087)
  spline S232 degree 2 poles (34.0734, 26.4087) (34.1335, 26.6352) (34.226, 26.8895) (34.471, 27.1021) (34.6928, 27.1021) knots 0 0 0 1 2 3 3 3
  spline S233 degree 2 poles (34.6928, 27.1021) (34.9193, 27.1021) (35.2522, 26.7878) (35.2522, 26.5751) knots 0 0 0 1 2 2 2
  spline S234 degree 2 poles (35.2522, 26.5751) (35.2522, 26.3995) (35.1181, 26.0297) knots 0 0 0 1 1 1
  line L102 (35.1181, 26.0297) -> (34.2352, 23.4365)
  spline S235 degree 2 poles (34.2352, 23.4365) (34.1381, 23.173) (34.0041, 22.854) (33.699, 22.5952) (33.4309, 22.5952) knots 0 0 0 1 2 3 3 3
  spline S236 degree 2 poles (33.4309, 22.5952) (33.1536, 22.5952) (32.8392, 22.8679) (32.6959, 23.2516) (32.622, 23.5058) knots 0 0 0 1 2 3 3 3
  line L103 (32.622, 23.5058) -> (32.0858, 25.5536)
  line L104 (32.0858, 25.5536) -> (31.568, 23.5058)
  spline S237 degree 2 poles (31.568, 23.5058) (31.4525, 23.0851) (31.152, 22.5952) (30.7591, 22.5952) knots 0 0 0 1 2 2 2
  spline S238 degree 2 poles (30.7591, 22.5952) (30.5603, 22.5952) (30.2784, 22.7523) (30.0935, 23.0343) (29.9779, 23.3579) (29.9317, 23.4919) knots 0 0 0 1 2 3 4 4 4
  line L105 (29.9317, 23.4919) -> (29.0719, 26.0297)
  spline S239 degree 2 poles (29.0719, 26.0297) (28.9332, 26.4226) (28.9332, 26.5751) knots 0 0 0 1 1 1
  spline S240 degree 2 poles (28.9332, 26.5751) (28.9332, 26.7831) (29.2522, 27.1021) (29.4925, 27.1021) knots 0 0 0 1 2 2 2
  spline S241 degree 2 poles (29.4925, 27.1021) (29.8022, 27.1021) (30.0195, 26.7508) (30.1304, 26.3764) knots 0 0 0 1 2 2 2
  line L106 (36.1027, 27.0096) -> (36.1351, 27.0096)
  line L107 (36.1351, 27.0096) -> (36.1351, 27.5736)
  spline S242 degree 2 poles (36.1351, 27.5736) (36.1351, 27.8371) (36.1628, 28.1468) (36.2552, 28.2993) knots 0 0 0 1 2 2 2
  spline S243 degree 2 poles (36.2552, 28.2993) (36.3061, 28.3964) (36.5834, 28.5536) (36.7499, 28.5536) knots 0 0 0 1 2 2 2
  spline S244 degree 2 poles (36.7499, 28.5536) (36.9856, 28.5536) (37.1751, 28.3779) knots 0 0 0 1 1 1
  spline S245 degree 2 poles (37.1751, 28.3779) (37.3046, 28.2577) (37.3693, 27.9295) (37.3693, 27.6568) knots 0 0 0 1 2 2 2
  line L108 (37.3693, 27.6568) -> (37.3693, 27.0096)
  line L109 (37.3693, 27.0096) -> (37.679, 27.0096)
  spline S246 degree 2 poles (37.679, 27.0096) (37.9378, 27.0096) (38.2291, 26.7462) (38.2291, 26.5474) knots 0 0 0 1 2 2 2
  spline S247 degree 2 poles (38.2291, 26.5474) (38.2291, 26.2793) (37.8223, 26.0759) (37.4848, 26.0759) knots 0 0 0 1 2 2 2
  line L110 (37.4848, 26.0759) -> (37.3693, 26.0759)
  line L111 (37.3693, 26.0759) -> (37.3693, 24.1899)
  spline S248 degree 2 poles (37.3693, 24.1899) (37.3693, 23.9403) (37.4016, 23.6999) (37.5126, 23.5798) (37.6466, 23.5798) knots 0 0 0 1 2 3 3 3
  spline S249 degree 2 poles (37.6466, 23.5798) (37.7344, 23.5798) (38.058, 23.6445) (38.1505, 23.6445) knots 0 0 0 1 2 2 2
  spline S250 degree 2 poles (38.1505, 23.6445) (38.3169, 23.6445) (38.5711, 23.3902) (38.5711, 23.21) knots 0 0 0 1 2 2 2
  spline S251 degree 2 poles (38.5711, 23.21) (38.5711, 22.9002) (37.9425, 22.5952) (37.397, 22.5952) knots 0 0 0 1 2 2 2
  spline S252 degree 2 poles (37.397, 22.5952) (36.87, 22.5952) (36.3061, 22.9603) (36.1351, 23.5982) (36.1351, 24.1067) knots 0 0 0 1 2 3 3 3
  line L112 (36.1351, 24.1067) -> (36.1351, 26.0759)
  line L113 (36.1351, 26.0759) -> (36.0796, 26.0759)
  spline S253 degree 2 poles (36.0796, 26.0759) (35.8115, 26.0759) (35.5203, 26.3394) (35.5203, 26.5474) knots 0 0 0 1 2 2 2
  spline S254 degree 2 poles (35.5203, 26.5474) (35.5203, 26.7508) (35.8254, 27.0096) (36.1027, 27.0096) knots 0 0 0 1 2 2 2
  line L114 (40.0087, 26.4226) -> (40.0087, 26.3764)
  spline S255 degree 2 poles (40.0087, 26.3764) (40.1705, 26.7277) (40.8546, 27.0929) (41.2891, 27.0929) knots 0 0 0 1 2 2 2
  spline S256 degree 2 poles (41.2891, 27.0929) (41.8022, 27.0929) (42.6759, 26.5566) (43.1751, 25.5443) (43.1751, 24.8602) knots 0 0 0 1 2 3 3 3
  spline S257 degree 2 poles (43.1751, 24.8602) (43.1751, 24.3517) (42.8885, 23.4965) (42.3801, 22.9095) (41.6867, 22.5952) (41.2891, 22.5952) knots 0 0 0 1 2 3 4 4 4
  spline S258 degree 2 poles (41.2891, 22.5952) (40.8038, 22.5952) (40.152, 22.9788) (40.0087, 23.3163) knots 0 0 0 1 2 2 2
  line L115 (40.0087, 23.3163) -> (40.0087, 21.7955)
  spline S259 degree 2 poles (40.0087, 21.7955) (40.0087, 21.0096) (39.4124, 21.0096) knots 0 0 0 1 1 1
  spline S260 degree 2 poles (39.4124, 21.0096) (39.0565, 21.0096) (38.83, 21.4349) (38.83, 21.8047) knots 0 0 0 1 2 2 2
  line L116 (38.83, 21.8047) -> (38.83, 26.4133)
  spline S261 degree 2 poles (38.83, 26.4133) (38.83, 26.7508) (39.1397, 27.1021) (39.4124, 27.1021) knots 0 0 0 1 2 2 2
  spline S262 degree 2 poles (39.4124, 27.1021) (39.6759, 27.1021) (40.0087, 26.7415) (40.0087, 26.4226) knots 0 0 0 1 2 2 2
  spline S263 degree 2 poles (41.9363, 24.8694) (41.9363, 25.2716) (41.6959, 25.8402) (41.2753, 26.1406) (41.0257, 26.1406) knots 0 0 0 1 2 3 3 3
  spline S264 degree 2 poles (41.0257, 26.1406) (40.6235, 26.1406) (40.0596, 25.4935) (40.0596, 24.8509) knots 0 0 0 1 2 2 2
  spline S265 degree 2 poles (40.0596, 24.8509) (40.0596, 24.2361) (40.6189, 23.5798) (41.0257, 23.5798) knots 0 0 0 1 2 2 2
  spline S266 degree 2 poles (41.0257, 23.5798) (41.266, 23.5798) (41.6774, 23.8617) (41.9363, 24.4442) (41.9363, 24.8694) knots 0 0 0 1 2 3 3 3
  line L117 (45.1998, 24.2223) -> (45.1998, 23.3301)
  spline S267 degree 2 poles (45.1998, 23.3301) (45.1998, 22.9696) (44.8485, 22.5952) (44.5757, 22.5952) knots 0 0 0 1 2 2 2
  spline S268 degree 2 poles (44.5757, 22.5952) (44.3076, 22.5952) (43.9656, 22.9742) (43.9656, 23.3301) knots 0 0 0 1 2 2 2
  line L118 (43.9656, 23.3301) -> (43.9656, 26.3024)
  spline S269 degree 2 poles (43.9656, 26.3024) (43.9656, 27.1021) (44.5711, 27.1021) knots 0 0 0 1 1 1
  spline S270 degree 2 poles (44.5711, 27.1021) (44.8808, 27.1021) (45.1489, 26.7138) (45.1536, 26.4411) knots 0 0 0 1 2 2 2
  spline S271 degree 2 poles (45.1536, 26.4411) (45.209, 26.7369) (45.6435, 27.1021) (46.0133, 27.1021) knots 0 0 0 1 2 2 2
  spline S272 degree 2 poles (46.0133, 27.1021) (46.3693, 27.1021) (47.0673, 26.7323) (47.0673, 26.4087) knots 0 0 0 1 2 2 2
  spline S273 degree 2 poles (47.0673, 26.4087) (47.0673, 26.1776) (46.7483, 25.8771) (46.5588, 25.8771) knots 0 0 0 1 2 2 2
  spline S274 degree 2 poles (46.5588, 25.8771) (46.4848, 25.8771) (46.0364, 26.0204) (45.8747, 26.0204) knots 0 0 0 1 2 2 2
  spline S275 degree 2 poles (45.8747, 26.0204) (45.6713, 26.0204) (45.4124, 25.8078) (45.2599, 25.3548) (45.1998, 24.7076) (45.1998, 24.2223) knots 0 0 0 1 2 3 4 4 4
  line L119 (48.7961, 26.418) -> (48.7961, 23.3301)
  spline S276 degree 2 poles (48.7961, 23.3301) (48.7961, 22.9742) (48.4448, 22.5952) (48.172, 22.5952) knots 0 0 0 1 2 2 2
  spline S277 degree 2 poles (48.172, 22.5952) (47.8993, 22.5952) (47.5619, 22.9835) (47.5619, 23.3301) knots 0 0 0 1 2 2 2
  line L120 (47.5619, 23.3301) -> (47.5619, 26.3856)
  spline S278 degree 2 poles (47.5619, 26.3856) (47.5619, 26.7323) (47.8993, 27.1021) (48.172, 27.1021) knots 0 0 0 1 2 2 2
  spline S279 degree 2 poles (48.172, 27.1021) (48.4448, 27.1021) (48.7961, 26.7323) (48.7961, 26.418) knots 0 0 0 1 2 2 2
  spline S280 degree 2 poles (48.1859, 27.4395) (47.9317, 27.4395) (47.5619, 27.7585) (47.5619, 28.0451) knots 0 0 0 1 2 2 2
  spline S281 degree 2 poles (47.5619, 28.0451) (47.5619, 28.3086) (47.9363, 28.646) (48.1859, 28.646) knots 0 0 0 1 2 2 2
  spline S282 degree 2 poles (48.1859, 28.646) (48.4217, 28.646) (48.7961, 28.3363) (48.7961, 28.0451) knots 0 0 0 1 2 2 2
  spline S283 degree 2 poles (48.7961, 28.0451) (48.7961, 27.7631) (48.4309, 27.4395) (48.1859, 27.4395) knots 0 0 0 1 2 2 2
  line L121 (50.9224, 26.4365) -> (50.9224, 26.3902)
  spline S284 degree 2 poles (50.9224, 26.3902) (51.0611, 26.7369) (51.7683, 27.1021) (52.226, 27.1021) knots 0 0 0 1 2 2 2
  spline S285 degree 2 poles (52.226, 27.1021) (52.6697, 27.1021) (53.377, 26.7138) (53.5526, 26.3579) knots 0 0 0 1 2 2 2
  spline S286 degree 2 poles (53.5526, 26.3579) (53.6636, 26.1499) (53.7283, 25.6737) (53.7283, 25.3178) knots 0 0 0 1 2 2 2
  line L122 (53.7283, 25.3178) -> (53.7283, 23.3301)
  spline S287 degree 2 poles (53.7283, 23.3301) (53.7283, 22.9742) (53.3908, 22.5952) (53.1181, 22.5952) knots 0 0 0 1 2 2 2
  spline S288 degree 2 poles (53.1181, 22.5952) (52.8408, 22.5952) (52.4987, 22.9835) (52.4987, 23.3301) knots 0 0 0 1 2 2 2
  line L123 (52.4987, 23.3301) -> (52.4987, 25.1098)
  spline S289 degree 2 poles (52.4987, 25.1098) (52.4987, 25.6183) (52.2352, 26.1175) (51.8469, 26.1175) knots 0 0 0 1 2 2 2
  spline S290 degree 2 poles (51.8469, 26.1175) (51.5881, 26.1175) (51.1628, 25.8078) (51.0472, 25.4981) knots 0 0 0 1 2 2 2
  spline S291 degree 2 poles (51.0472, 25.4981) (50.9871, 25.3132) (50.9871, 24.6707) knots 0 0 0 1 1 1
  line L124 (50.9871, 24.6707) -> (50.9871, 23.3301)
  spline S292 degree 2 poles (50.9871, 23.3301) (50.9871, 22.9696) (50.6405, 22.5952) (50.3631, 22.5952) knots 0 0 0 1 2 2 2
  spline S293 degree 2 poles (50.3631, 22.5952) (50.095, 22.5952) (49.7529, 22.9835) (49.7529, 23.3301) knots 0 0 0 1 2 2 2
  line L125 (49.7529, 23.3301) -> (49.7529, 26.418)
  spline S294 degree 2 poles (49.7529, 26.418) (49.7529, 26.7508) (50.0626, 27.1021) (50.3307, 27.1021) knots 0 0 0 1 2 2 2
  spline S295 degree 2 poles (50.3307, 27.1021) (50.4972, 27.1021) (50.7653, 26.9449) (50.9224, 26.6398) (50.9224, 26.4365) knots 0 0 0 1 2 3 3 3
  line L126 (54.8747, 27.0096) -> (54.907, 27.0096)
  line L127 (54.907, 27.0096) -> (54.907, 27.5736)
  spline S296 degree 2 poles (54.907, 27.5736) (54.907, 27.8371) (54.9348, 28.1468) (55.0272, 28.2993) knots 0 0 0 1 2 2 2
  spline S297 degree 2 poles (55.0272, 28.2993) (55.0781, 28.3964) (55.3554, 28.5536) (55.5218, 28.5536) knots 0 0 0 1 2 2 2
  spline S298 degree 2 poles (55.5218, 28.5536) (55.7576, 28.5536) (55.9471, 28.3779) knots 0 0 0 1 1 1
  spline S299 degree 2 poles (55.9471, 28.3779) (56.0765, 28.2577) (56.1412, 27.9295) (56.1412, 27.6568) knots 0 0 0 1 2 2 2
  line L128 (56.1412, 27.6568) -> (56.1412, 27.0096)
  line L129 (56.1412, 27.0096) -> (56.4509, 27.0096)
  spline S300 degree 2 poles (56.4509, 27.0096) (56.7098, 27.0096) (57.001, 26.7462) (57.001, 26.5474) knots 0 0 0 1 2 2 2
  spline S301 degree 2 poles (57.001, 26.5474) (57.001, 26.2793) (56.5942, 26.0759) (56.2568, 26.0759) knots 0 0 0 1 2 2 2
  line L130 (56.2568, 26.0759) -> (56.1412, 26.0759)
  line L131 (56.1412, 26.0759) -> (56.1412, 24.1899)
  spline S302 degree 2 poles (56.1412, 24.1899) (56.1412, 23.9403) (56.1736, 23.6999) (56.2845, 23.5798) (56.4186, 23.5798) knots 0 0 0 1 2 3 3 3
  spline S303 degree 2 poles (56.4186, 23.5798) (56.5064, 23.5798) (56.83, 23.6445) (56.9224, 23.6445) knots 0 0 0 1 2 2 2
  spline S304 degree 2 poles (56.9224, 23.6445) (57.0888, 23.6445) (57.3431, 23.3902) (57.3431, 23.21) knots 0 0 0 1 2 2 2
  spline S305 degree 2 poles (57.3431, 23.21) (57.3431, 22.9002) (56.7144, 22.5952) (56.169, 22.5952) knots 0 0 0 1 2 2 2
  spline S306 degree 2 poles (56.169, 22.5952) (55.642, 22.5952) (55.0781, 22.9603) (54.907, 23.5982) (54.907, 24.1067) knots 0 0 0 1 2 3 3 3
  line L132 (54.907, 24.1067) -> (54.907, 26.0759)
  line L133 (54.907, 26.0759) -> (54.8515, 26.0759)
  spline S307 degree 2 poles (54.8515, 26.0759) (54.5834, 26.0759) (54.2922, 26.3394) (54.2922, 26.5474) knots 0 0 0 1 2 2 2
  spline S308 degree 2 poles (54.2922, 26.5474) (54.2922, 26.7508) (54.5973, 27.0096) (54.8747, 27.0096) knots 0 0 0 1 2 2 2
  spline S309 degree 2 poles (59.3539, 26.3209) (59.6821, 26.3209) (60.1536, 26.6999) (60.1536, 27.0605) knots 0 0 0 1 2 2 2
  spline S310 degree 2 poles (60.1536, 27.0605) (60.1536, 27.324) (59.7838, 27.7123) (59.4694, 27.7123) knots 0 0 0 1 2 2 2
  spline S311 degree 2 poles (59.4694, 27.7123) (59.2475, 27.7123) (58.9702, 27.5921) (58.813, 27.4026) (58.6374, 27.0235) (58.5865, 26.9126) knots 0 0 0 1 2 3 4 4 4
  spline S312 degree 2 poles (58.5865, 26.9126) (58.5357, 26.797) (58.2907, 26.6861) (58.1381, 26.6861) knots 0 0 0 1 2 2 2
  spline S313 degree 2 poles (58.1381, 26.6861) (57.944, 26.6861) (57.6343, 26.9912) (57.6343, 27.2361) knots 0 0 0 1 2 2 2
  spline S314 degree 2 poles (57.6343, 27.2361) (57.6343, 27.4627) (57.8978, 27.9388) (58.397, 28.364) (59.1274, 28.6229) (59.5757, 28.6229) knots 0 0 0 1 2 3 4 4 4
  spline S315 degree 2 poles (59.5757, 28.6229) (59.9687, 28.6229) (60.625, 28.4056) (61.115, 27.9896) (61.3646, 27.4442) (61.3646, 27.1298) knots 0 0 0 1 2 3 4 4 4
  spline S316 degree 2 poles (61.3646, 27.1298) (61.3646, 26.7184) (61.0041, 26.1221) (60.7083, 25.9234) knots 0 0 0 1 2 2 2
  spline S317 degree 2 poles (60.7083, 25.9234) (60.981, 25.8124) (61.4201, 25.3687) (61.642, 24.8278) (61.642, 24.5135) knots 0 0 0 1 2 3 3 3
  spline S318 degree 2 poles (61.642, 24.5135) (61.642, 24.1437) (61.3415, 23.4457) (60.7637, 22.9002) (59.9687, 22.5952) (59.4925, 22.5952) knots 0 0 0 1 2 3 4 4 4
  spline S319 degree 2 poles (59.4925, 22.5952) (59.0025, 22.5952) (58.226, 22.9465) (57.7267, 23.4734) (57.4679, 24.042) (57.4679, 24.2361) knots 0 0 0 1 2 3 4 4 4
  spline S320 degree 2 poles (57.4679, 24.2361) (57.4679, 24.4996) (57.8099, 24.8232) (58.0642, 24.8232) knots 0 0 0 1 2 2 2
  spline S321 degree 2 poles (58.0642, 24.8232) (58.1982, 24.8232) (58.4432, 24.6614) (58.4895, 24.5181) knots 0 0 0 1 2 2 2
  spline S322 degree 2 poles (58.4895, 24.5181) (58.6836, 24.0189) (59.1135, 23.5289) (59.5018, 23.5289) knots 0 0 0 1 2 2 2
  spline S323 degree 2 poles (59.5018, 23.5289) (59.7237, 23.5289) (60.1304, 23.7462) (60.4032, 24.1807) (60.4032, 24.4673) knots 0 0 0 1 2 3 3 3
  spline S324 degree 2 poles (60.4032, 24.4673) (60.4032, 24.8925) (59.9455, 25.364) (59.5388, 25.364) knots 0 0 0 1 2 2 2
  spline S325 degree 2 poles (59.5388, 25.364) (59.4694, 25.364) (59.1412, 25.3317) (59.0858, 25.3317) knots 0 0 0 1 2 2 2